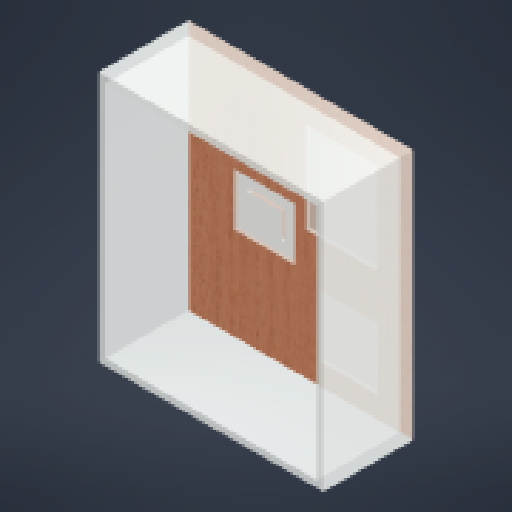
# Autodesk Inventor part: Shooting Mechanism Box
Saved by Autodesk Inventor 2026.2 (Build 302298000, 298)
## iProperties
Created: 2026-04-11
Part Number: Shooting Mechanism Box
Material: Glass
Document SubType Name: Modeling
Designer: abdul
Density: 2.18 g/cm^3
Appearance: Clear
Author: abdul
Autodesk Inventor part; units mm, degrees
ref_plane "YZ Plane" through (0, 0, 0) normal (1, 0, 0) x (0, 1, 0)
ref_plane "XZ Plane" through (0, 0, 0) normal (0, 1, 0) x (-1, 0, 0)
ref_plane "XY Plane" through (0, 0, 0) normal (0, 0, 1) x (1, 0, 0)
sketch "Sketch1" plane through (0, 0, 0) normal (0, 0, 1) x (1, 0, 0)
  line L0 (90, -90) -> (-70, -90)
  line L1 (-70, -90) -> (-70, 90)
  line L2 (-70, 90) -> (90, 90)
  line L3 (90, 90) -> (90, -90)
  line L4 (95, 95) -> (-75, 95)
  line L5 (-75, 95) -> (-75, -95)
  line L6 (-75, -95) -> (95, -95)
  line L7 (95, -95) -> (95, 95)
  point P0 (0, 0)
  dimension "d45" = 180
  dimension "d46" = 5
  dimension "d61" = 70
  dimension "d62" = 90
  dimension "d63" = 5
  constraints: 16 end point, 3 parallel, 2 perpendicular, 1 horizontal, 1 vertical, 2 other
  measures "d45" distance of L0.end L1.end
  measures "d46" distance between parallel lines of L2 L4
  measures "d61" distance from line of L1 point (0, 0)
  measures "d62" distance from line of point (0, 0) L3
  measures "d63" distance between parallel lines of L7 L3
extrude "Extrusion1" add sketch "Sketch1" along normal blind 68
extrude "Extrusion2" add sketch "Sketch1" along normal blind 5 contours L0 L1 L2 L3
sketch "Sketch2" plane through (0, 0, 5) normal (0, 0, 1) x (1, 0, 0)
  line L0 (29.7141, -27.0003) -> (73.7141, -27.0003)
  line L1 (73.7141, -27.0003) -> (73.7141, -74.0003)
  line L2 (73.7141, -74.0003) -> (29.7141, -74.0003)
  line L3 (29.7141, -74.0003) -> (29.7141, -27.0003)
  circle A0 centre (0, 0) radius 150 construction
  line L4 (72.9434, 76.0673) -> (72.9434, 7.0673)
  line L5 (72.9434, 7.0673) -> (18.9434, 7.0673)
  line L6 (18.9434, 7.0673) -> (18.9434, 76.0673)
  line L7 (18.9434, 76.0673) -> (72.9434, 76.0673)
  line L8 (45.9434, 76.0673) -> (45.9434, 7.0673) construction
  line L9 (-70, -90) -> (90, -90)
  line L10 (90, -90) -> (90, 90)
  line L11 (90, 90) -> (-70, 90)
  line L12 (-70, 90) -> (-70, -90)
  line L13 (90, 90) -> (90, -90) projected
  line L14 (-25.5, -10) -> (0.5, -10)
  line L15 (0.5, -10) -> (0.5, 10)
  line L16 (0.5, 10) -> (-25.5, 10)
  line L17 (-25.5, 10) -> (-25.5, -10)
  line L18 (-35.5, -20) -> (10.5, -20)
  line L19 (10.5, -20) -> (10.5, 20)
  line L20 (10.5, 20) -> (-35.5, 20)
  line L21 (-35.5, 20) -> (-35.5, -20)
  point P0 (51.7141, -50.5003)
  point P1 (73.7141, -50.5003)
  point P2 (51.7141, -27.0003)
  point P3 (45.9434, 41.5673)
  dimension "d6" = 47
  dimension "d7" = 44
  dimension "d8" = 54
  dimension "d9" = 69
  dimension "d47" = 160
  dimension "d48" = 160
  dimension "d54" = 26
  dimension "d55" = 20
  dimension "d56" = 46
  dimension "d57" = 40
  dimension "d58" = 0.5
  dimension "d59" = 10
  dimension "d60" = 10
  constraints: 42 end point, 8 parallel, 7 perpendicular, 5 midpoint, 4 horizontal, 1 horizontal alignment, 1 vertical alignment
  measures "d6" distance of L2.end L0.start
  measures "d7" distance of L1.end L2.end
  measures "d8" distance of L6.end L4.start
  measures "d9" distance of L4.start L4.end
  measures "d47" distance of L11.end L10.end
  measures "d54" distance of L16.end L15.end
  measures "d55" distance of L15.end L14.end
  measures "d56" distance of L20.end L19.end
  measures "d57" distance of L19.end L18.end
  measures "d58" distance from line of L15 A0.centre
  measures "d59" distance between parallel lines of L21 L17
  measures "d60" distance between parallel lines of L20 L16
extrude "Extrusion3" cut sketch "Sketch2" against normal blind 1.5 contours L0 L1 L2 L3 | L4 L5 L6 L7
extrude "Extrusion4" cut sketch "Sketch2" against normal blind 3 contours L0 L1 L2 L3 | L4 L5 L6 L7 | L21 L20 L19 L18
body "Solid1"
